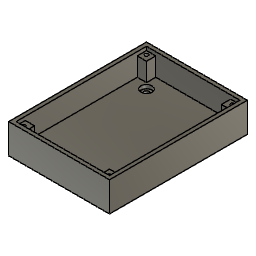
Halterung Platine v2 (Autodesk Fusion 360 design; units mm, degrees)
Autodesk Fusion 360 part; units mm, degrees
sketch "Skizze1" plane through (0, 0, 0) normal (0, 0, 1) x (1, 0, 0)
  line L0 (-27.25, 37.25) -> (27.25, 37.25)
  line L1 (27.25, 37.25) -> (27.25, -37.25)
  line L2 (27.25, -37.25) -> (-27.25, -37.25)
  line L3 (-27.25, -37.25) -> (-27.25, 37.25)
  line L4 (-27.25, 37.25) -> (27.25, -37.25) construction
  line L5 (27.25, 37.25) -> (-27.25, -37.25) construction
  dimension "d1" = 54.5
  dimension "d2" = 74.5
  constraint horizontal L0
  constraint perpendicular L0 L1
  constraint parallel L0 L2
  constraint parallel L1 L3
  constraint coincident L4 origin
  constraint coincident L5 origin
  measures "d1" distance of L1.end L2.end
  measures "d2" distance of L0.end L1.end
extrude "Extrusion1" add sketch "Skizze1" along normal blind 20
shell "Schale1" thickness 2 removed faces 1 at (-9.0833, 12.4167, 20)
extrude "Extrusion2" cut 1 faces at (26.5833, -11.75, 20) along direction (0, 0, -1) blind 6
sketch "Skizze2" plane through (0, 0, 2) normal (0, 0, 1) x (-1, 0, 0)
  line L0 (25.25, 35.25) -> (-25.25, 35.25)
  line L1 (-25.25, 35.25) -> (-25.25, -35.25)
  line L2 (-25.25, -35.25) -> (25.25, -35.25)
  line L3 (25.25, -35.25) -> (25.25, 35.25)
  line L4 (25.25, -35.25) -> (20.25, -35.25)
  line L5 (20.25, -35.25) -> (20.25, -30.25)
  line L6 (20.25, -30.25) -> (25.25, -30.25)
  line L7 (25.25, -30.25) -> (25.25, -35.25)
  line L8 (-25.25, -35.25) -> (-20.25, -35.25)
  line L9 (-20.25, -35.25) -> (-20.25, -30.25)
  line L10 (-20.25, -30.25) -> (-25.25, -30.25)
  line L11 (-25.25, -30.25) -> (-25.25, -35.25)
  line L12 (25.25, 35.25) -> (20.25, 35.25)
  line L13 (20.25, 35.25) -> (20.25, 30.25)
  line L14 (20.25, 30.25) -> (25.25, 30.25)
  line L15 (25.25, 30.25) -> (25.25, 35.25)
  line L16 (-25.25, 35.25) -> (-20.25, 35.25)
  line L17 (-20.25, 35.25) -> (-20.25, 30.25)
  line L18 (-20.25, 30.25) -> (-25.25, 30.25)
  line L19 (-25.25, 30.25) -> (-25.25, 35.25)
  dimension "d8" = 5
  dimension "d9" = 5
  dimension "d10" = 5
  dimension "d11" = 5
  dimension "d12" = 5
  dimension "d13" = 5
  dimension "d14" = 5
  dimension "d15" = 5
  constraint horizontal L4
  constraint vertical L5
  constraint horizontal L6
  constraint vertical L7
  constraint coincident L2.end L3.start
  constraint horizontal L8
  constraint vertical L9
  constraint horizontal L10
  constraint vertical L11
  constraint coincident L1.end L2.start
  constraint horizontal L12
  constraint vertical L13
  constraint horizontal L14
  constraint vertical L15
  constraint coincident L0.start L3.end
  constraint horizontal L16
  constraint vertical L17
  constraint horizontal L18
  constraint vertical L19
  constraint coincident L0.end L1.start
  measures "d8" distance of L2.end L4.end
  measures "d9" distance of L2.end L6.end
  measures "d10" distance of L1.end L8.end
  measures "d11" distance of L1.end L10.end
  measures "d12" distance of L0.start L12.end
  measures "d13" distance of L0.start L14.end
  measures "d14" distance of L0.end L16.end
  measures "d15" distance of L0.end L18.end
extrude "Extrusion3" add sketch "Skizze2" along normal blind 10 contours L0 L3 L12 L13 L14 L15 | L0 L1 L16 L17 L18 L19 | L2 L3 L4 L5 L6 L7 | L1 L2 L8 L9 L10 L11
sketch "Skizze3" plane through (0, 0, 12) normal (0, 0, 1) x (-1, 0, 0)
  line L0 (25.25, -30.25) -> (20.25, -30.25)
  line L1 (20.25, -30.25) -> (20.25, -35.25)
  line L2 (20.25, -35.25) -> (25.25, -35.25)
  line L3 (25.25, -35.25) -> (25.25, -30.25)
  circle A0 centre (23.25, -33.25) radius 1
  circle A1 centre (-23.25, -33.25) radius 1
  circle A2 centre (23.25, 33.25) radius 1
  circle A3 centre (-23.25, 33.25) radius 1
  dimension "d20" = 2
  measures "d20" diameter of A0
extrude "Extrusion4" cut sketch "Skizze3" against normal blind 12 contours A0 | A1 | A2 | A3
extrude "Extrusion5" add 1 faces at (7.518, -10.8051, 0) along direction (0, 0, -1) blind 2
move_body "Verschieben1" bodies 1 to x (1, 0, 0) y (0, 1, 0) z (0, 0, 1) at (0, 0, 2)
sketch "Skizze4" plane through (0, 0, 4) normal (0, 0, 1) x (-1, 0, 0)
  line L0 (25.25, 30.25) -> (20.25, 30.25)
  line L1 (20.25, 30.25) -> (20.25, 35.25)
  line L2 (20.25, 35.25) -> (-20.25, 35.25)
  line L3 (-20.25, 35.25) -> (-20.25, 30.25)
  line L4 (-20.25, 30.25) -> (-25.25, 30.25)
  line L5 (-25.25, 30.25) -> (-25.25, -30.25)
  line L6 (-25.25, -30.25) -> (-20.25, -30.25)
  line L7 (-20.25, -30.25) -> (-20.25, -35.25)
  line L8 (-20.25, -35.25) -> (20.25, -35.25)
  line L9 (25.25, -30.25) -> (25.25, 30.25)
  circle A0 centre (17.25, -27.25) radius 3
  circle A1 centre (-17.25, -27.25) radius 3
  circle A2 centre (17.25, 27.25) radius 3
  circle A3 centre (-17.25, 27.25) radius 3
  dimension "d27" = 6
  measures "d27" diameter of A0
extrude "Extrusion6" cut sketch "Skizze4" against normal blind 2
sketch "Skizze5" plane through (0, 0, 2) normal (0, 0, 1) x (-1, 0, 0)
  circle A0 centre (17.25, -27.25) radius 3
  circle A1 centre (17.25, -27.25) radius 1.65
  circle A2 centre (-17.25, -27.25) radius 1.65
  circle A3 centre (17.25, 27.25) radius 1.65
  circle A4 centre (-17.25, 27.25) radius 1.65
  point P0 (-17.25, -27.25)
  point P1 (17.25, 27.25)
  point P2 (-17.25, 27.25)
  dimension "d30" = 3.3
  constraint concentric A0 A1
  measures "d30" diameter of A1
extrude "Extrusion7" cut sketch "Skizze5" against normal blind 2 contours A1 | A2 | A3 | A4
